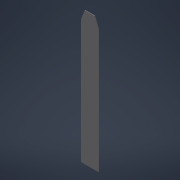
# Autodesk Inventor part: PlanchaHorqSup
Saved by Autodesk Inventor 2022 (Build 260153000, 153)
## iProperties
Created: 2021-09-29
Part Number: PlanchaHorqSup
Material: Steel, Mild, Welded
Document SubType Name: Sheet Metal
Designer: Andres
Mass: 9380.75 g
Surface Area: 4929.77 cm^2
Volume: 1195 cm^3
Density: 7.85 g/cm^3
Sheet Metal Rule: Default_mm
Appearance: Weld - Steel Mild
Author: Andres
Autodesk Inventor part; units mm, degrees
ref_plane "YZ Plane" through (0, 0, 0) normal (1, 0, 0) x (0, 1, 0)
ref_plane "XZ Plane" through (0, 0, 0) normal (0, 1, 0) x (-1, 0, 0)
ref_plane "XY Plane" through (0, 0, 0) normal (0, 0, 1) x (1, 0, 0)
sketch "Sketch1" plane through (0, 0, 0) normal (0, 0, 1) x (1, 0, 0)
  line L0 (15, 1250) -> (15, 0)
  line L1 (195, 1250) -> (195, 0)
  line L2 (15, 0) -> (195, 0)
  line L3 (15, 1250) -> (55, 1350)
  line L4 (55, 1350) -> (155, 1350)
  line L5 (155, 1350) -> (195, 1250)
  point P0 (0, 0)
extrude "Plate1" add sketch "Sketch1" along normal blind 5
equation "\"d0\" = Thickness"
equation "\"BendRadius\" = Thickness"
equation "\"BendReliefWidth\" = Thickness"
equation "\"BendReliefDepth\" = 0.5 * Thickness"
equation "\"TransitionRadius\" = BendRadius"
equation "\"JacobiRadiusSize\" = BendRadius"
equation "\"GapSize\" = Thickness"
equation "\"Thickness\" = 5"
body "Solid1"
